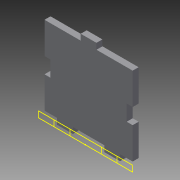
# Autodesk Inventor part: sideR
Saved by Autodesk Inventor 2015 SP1 (Build 190203100, 203)
## iProperties
Created: 2016-04-13
Part Number: sideR
Material: Generic
Document SubType Name: Modeling
Designer: tuttlem
Density: 1 g/cm^3
Appearance: Default
Author: tuttlem
Autodesk Inventor part; units mm, degrees
ref_plane "YZ Plane" through (0, 0, 0) normal (1, 0, 0) x (0, 1, 0)
ref_plane "XZ Plane" through (0, 0, 0) normal (0, 1, 0) x (-1, 0, 0)
ref_plane "XY Plane" through (0, 0, 0) normal (0, 0, 1) x (1, 0, 0)
sketch "Sketch1" plane through (0, 0, 0) normal (0, 0, 1) x (1, 0, 0)
  line L0 (-38.1, 0) -> (38.1, 0) projected
  line L1 (38.1, 0) -> (38.1, 4.826) projected
  line L2 (-38.1, 4.826) -> (38.1, 4.826) projected
  line L3 (-38.1, 0) -> (-38.1, 4.826) projected
  line L4 (-25.4, 0) -> (-12.7, 0) projected
  line L5 (-25.4, 0) -> (-25.4, 4.826) projected
  line L6 (-12.7, 4.826) -> (-25.4, 4.826) projected
  line L7 (-12.7, 0) -> (-12.7, 4.826) projected
  line L8 (12.7, 0) -> (25.4, 0) projected
  line L9 (12.7, 0) -> (12.7, 4.826) projected
  line L10 (25.4, 4.826) -> (12.7, 4.826) projected
  line L11 (25.4, 0) -> (25.4, 4.826) projected
  point P0 (0, 0)
ref_plane "Work Plane1" through (-12.7, 0, -7.366) normal (0, 0, 1) x (1, 0, 0)
sketch "Sketch2" plane through (-12.7, 0, -7.366) normal (0, 0, 1) x (1, 0, 0)
  line L0 (0, 0) -> (-12.7, 0) projected
  line L1 (0, 0) -> (0, 4.826) projected
  line L2 (-12.7, 4.826) -> (0, 4.826) projected
  line L3 (-12.7, 0) -> (-12.7, 4.826) projected
  line L4 (-12.7, 0) -> (0, 0)
  line L5 (0, 0) -> (0, 4.826)
  line L6 (-12.7, 4.826) -> (-12.7, 0)
  line L7 (38.1, 0) -> (25.4, 0) projected
  line L8 (38.1, 0) -> (38.1, 4.826) projected
  line L9 (25.4, 4.826) -> (38.1, 4.826) projected
  line L10 (25.4, 0) -> (25.4, 4.826) projected
  line L11 (25.4, 0) -> (38.1, 0)
  line L12 (38.1, 0) -> (38.1, 4.826)
  line L13 (25.4, 4.826) -> (25.4, 0)
  line L14 (-18.034, 0) -> (-22.86, 0) projected
  line L15 (-18.034, 0) -> (-18.034, 4.826) projected
  line L16 (-22.86, 4.826) -> (-18.034, 4.826) projected
  line L17 (-22.86, 0) -> (-22.86, 4.826) projected
  line L18 (43.434, 0) -> (48.26, 0) projected
  line L19 (43.434, 0) -> (43.434, 4.826) projected
  line L20 (48.26, 4.826) -> (43.434, 4.826) projected
  line L21 (48.26, 0) -> (48.26, 4.826) projected
  line L22 (48.26, 68.326) -> (-22.86, 68.326)
  line L23 (-22.86, 42.926) -> (-18.034, 42.926)
  line L24 (-18.034, 42.926) -> (-18.034, 30.226)
  line L25 (-18.034, 30.226) -> (-22.86, 30.226)
  line L26 (48.26, 42.926) -> (43.434, 42.926)
  line L27 (43.434, 42.926) -> (43.434, 30.226)
  line L28 (43.434, 30.226) -> (48.26, 30.226)
  line L29 (-22.86, 68.326) -> (-22.86, 42.926)
  line L30 (-22.86, 30.226) -> (-22.86, 4.826)
  line L31 (48.26, 4.826) -> (48.26, 30.226)
  line L32 (48.26, 42.926) -> (48.26, 68.326)
  line L33 (-22.86, 4.826) -> (-12.7, 4.826)
  line L34 (0, 4.826) -> (25.4, 4.826)
  line L35 (38.1, 4.826) -> (48.26, 4.826)
  point P0 (12.7, 0)
  dimension "d0" = 63.5
  dimension "d2" = 12.7
  dimension "d3" = 25.4
  dimension "d5" = 4.826
  constraints: 41 end point, 10 parallel, 9 perpendicular, 6 horizontal, 1 point on line
  measures "d0" distance of L22.start L31.start
  measures "d2" distance of L23.end L24.end
  measures "d3" distance between parallel lines of L23 L22
  measures "d5" distance of L24.end L25.end
extrude "Extrusion1" add sketch "Sketch2" along normal blind 4.826 contours L0 L3 L2 L1 | L2 L33 L16 L30 L25 L24 L23 L29 L22 L32 L26 L27 L28 L31 L20 L35 L9 L34 | L9 L8 L7 L10
sketch "Sketch3" plane through (-12.7, 0, -2.54) normal (0, 0, 1) x (1, 0, 0)
  line L0 (48.26, 68.326) -> (-22.86, 68.326) projected
  line L1 (-22.86, 68.326) -> (-22.86, 42.926) projected
  line L2 (48.26, 68.326) -> (-22.86, 68.326) projected
  line L3 (6.35, 68.326) -> (19.05, 68.326)
  line L4 (19.05, 68.326) -> (19.05, 73.152)
  line L5 (19.05, 73.152) -> (6.35, 73.152)
  line L6 (6.35, 73.152) -> (6.35, 68.326)
  point P0 (12.7, 0)
  dimension "d8" = 12.7
  dimension "d9" = 4.826
  dimension "d10" = 29.21
  constraints: 8 end point, 2 parallel, 1 horizontal, 1 perpendicular, 1 point on line
  measures "d8" distance of L5.end L4.end
  measures "d9" distance of L4.end L3.end
  measures "d10" distance between parallel lines of L6 L1
extrude "Extrusion2" add sketch "Sketch3" against normal blind 4.826
sketch "Sketch4" plane through (-12.7, 0, -2.54) normal (0, 0, 1) x (1, 0, 0)
  line L0 (0, 4.826) -> (25.4, 4.826) projected
  line L1 (6.35, 4.826) -> (19.05, 4.826)
  line L2 (19.05, 4.826) -> (19.05, 11.176)
  line L3 (19.05, 11.176) -> (6.35, 11.176)
  line L4 (6.35, 11.176) -> (6.35, 4.826)
  line L5 (48.26, 4.826) -> (48.26, 30.226) projected
  point P0 (12.7, 0)
  dimension "d13" = 12.7
  dimension "d14" = 6.35
  dimension "d15" = 29.21
  constraints: 8 end point, 2 parallel, 1 horizontal, 1 perpendicular, 1 point on line
  measures "d13" distance of L3.end L2.end
  measures "d14" distance of L3.end L1.start
  measures "d15" distance between parallel lines of L5 L2
body "Solid1"
